Autodesk Fusion 360 part; units mm, degrees
(part 3 of 9)
  line L388 (-87.1879, -68.7148) -> (-81.5345, -68.7148) construction
  line L389 (-81.5345, -68.7148) -> (-81.5345, -58.1314) construction
  line L390 (-81.5345, -58.1314) -> (-87.1879, -58.1314) construction
  line L391 (-87.1879, -58.1314) -> (-87.1879, -68.7148) construction
  line L392 (-70.5192, -68.7148) -> (-65.7856, -68.7148) construction
  line L393 (-65.7856, -68.7148) -> (-65.7856, -58.1314) construction
  line L394 (-65.7856, -58.1314) -> (-70.5192, -58.1314) construction
  line L395 (-70.5192, -58.1314) -> (-70.5192, -68.7148) construction
  line L396 (-53.8504, -68.7148) -> (-48.7396, -68.7148) construction
  line L397 (-48.7396, -68.7148) -> (-48.7396, -58.1314) construction
  line L398 (-48.7396, -58.1314) -> (-53.8504, -58.1314) construction
  line L399 (-53.8504, -58.1314) -> (-53.8504, -68.7148) construction
  line L400 (-37.1817, -68.7148) -> (-30.2519, -68.7148) construction
  line L401 (-30.2519, -68.7148) -> (-30.2519, -58.1314) construction
  line L402 (-30.2519, -58.1314) -> (-37.1817, -58.1314) construction
  line L403 (-37.1817, -58.1314) -> (-37.1817, -68.7148) construction
  line L404 (-17.0129, -68.7148) -> (-16.0104, -68.7148) construction
  line L405 (-16.0104, -68.7148) -> (-16.0104, -58.1314) construction
  line L406 (-16.0104, -58.1314) -> (-17.0129, -58.1314) construction
  line L407 (-17.0129, -58.1314) -> (-17.0129, -68.7148) construction
  line L408 (-3.8442, -68.7148) -> (1.8092, -68.7148) construction
  line L409 (1.8092, -68.7148) -> (1.8092, -58.1314) construction
  line L410 (1.8092, -58.1314) -> (-3.8442, -58.1314) construction
  line L411 (-3.8442, -58.1314) -> (-3.8442, -68.7148) construction
  line L412 (12.8246, -68.7148) -> (19.5012, -68.7148) construction
  line L413 (19.5012, -68.7148) -> (19.5012, -58.1314) construction
  line L414 (19.5012, -58.1314) -> (12.8246, -58.1314) construction
  line L415 (12.8246, -58.1314) -> (12.8246, -68.7148) construction
  line L416 (29.4933, -68.7148) -> (36.5833, -68.7148) construction
  line L417 (36.5833, -68.7148) -> (36.5833, -58.1314) construction
  line L418 (36.5833, -58.1314) -> (29.4933, -58.1314) construction
  line L419 (29.4933, -58.1314) -> (29.4933, -68.7148) construction
  line L420 (46.1621, -68.7148) -> (52.8593, -68.7148) construction
  line L421 (52.8593, -68.7148) -> (52.8593, -58.1314) construction
  line L422 (52.8593, -58.1314) -> (46.1621, -58.1314) construction
  line L423 (46.1621, -58.1314) -> (46.1621, -68.7148) construction
  line L424 (62.8308, -68.7148) -> (68.7736, -68.7148) construction
  line L425 (68.7736, -68.7148) -> (68.7736, -58.1314) construction
  line L426 (68.7736, -58.1314) -> (62.8308, -58.1314) construction
  line L427 (62.8308, -58.1314) -> (62.8308, -68.7148) construction
  line L428 (79.4996, -68.7148) -> (85.5044, -68.7148) construction
  line L429 (85.5044, -68.7148) -> (85.5044, -58.1314) construction
  line L430 (85.5044, -58.1314) -> (79.4996, -58.1314) construction
  line L431 (79.4996, -58.1314) -> (79.4996, -68.7148) construction
  line L432 (96.1683, -68.7148) -> (102.5183, -68.7148) construction
  line L433 (102.5183, -68.7148) -> (102.5183, -58.1314) construction
  line L434 (102.5183, -58.1314) -> (96.1683, -58.1314) construction
  line L435 (96.1683, -58.1314) -> (96.1683, -68.7148) construction
  line L436 (-87.1879, -87.2148) -> (-81.1573, -87.2148) construction
  line L437 (-81.1573, -87.2148) -> (-81.1573, -76.6314) construction
  line L438 (-81.1573, -76.6314) -> (-87.1879, -76.6314) construction
  line L439 (-87.1879, -76.6314) -> (-87.1879, -87.2148) construction
  line L440 (-70.5192, -87.2148) -> (-64.8658, -87.2148) construction
  line L441 (-64.8658, -87.2148) -> (-64.8658, -76.6314) construction
  line L442 (-64.8658, -76.6314) -> (-70.5192, -76.6314) construction
  line L443 (-70.5192, -76.6314) -> (-70.5192, -87.2148) construction
  line L444 (-53.8504, -87.2148) -> (-47.1532, -87.2148) construction
  line L445 (-47.1532, -87.2148) -> (-47.1532, -76.6314) construction
  line L446 (-47.1532, -76.6314) -> (-53.8504, -76.6314) construction
  line L447 (-53.8504, -76.6314) -> (-53.8504, -87.2148) construction
  line L448 (-37.1817, -87.2148) -> (-31.2389, -87.2148) construction
  line L449 (-31.2389, -87.2148) -> (-31.2389, -76.6314) construction
  line L450 (-31.2389, -76.6314) -> (-37.1817, -76.6314) construction
  line L451 (-37.1817, -76.6314) -> (-37.1817, -87.2148) construction
  line L452 (-20.5129, -87.2148) -> (-14.4823, -87.2148) construction
  line L453 (-14.4823, -87.2148) -> (-14.4823, -76.6314) construction
  line L454 (-14.4823, -76.6314) -> (-20.5129, -76.6314) construction
  line L455 (-20.5129, -76.6314) -> (-20.5129, -87.2148) construction
  line L456 (-0.3442, -87.2148) -> (0.6584, -87.2148) construction
  line L457 (0.6584, -87.2148) -> (0.6584, -76.6314) construction
  line L458 (0.6584, -76.6314) -> (-0.3442, -76.6314) construction
  line L459 (-0.3442, -76.6314) -> (-0.3442, -87.2148) construction
  line L460 (12.8246, -87.2148) -> (18.7829, -87.2148) construction
  line L461 (18.7829, -87.2148) -> (18.7829, -76.6314) construction
  line L462 (18.7829, -76.6314) -> (12.8246, -76.6314) construction
  line L463 (12.8246, -76.6314) -> (12.8246, -87.2148) construction
  line L464 (29.4933, -87.2148) -> (35.4361, -87.2148) construction
  line L465 (35.4361, -87.2148) -> (35.4361, -76.6314) construction
  line L466 (35.4361, -76.6314) -> (29.4933, -76.6314) construction
  line L467 (29.4933, -76.6314) -> (29.4933, -87.2148) construction
  line L468 (46.1621, -87.2148) -> (52.8387, -87.2148) construction
  line L469 (52.8387, -87.2148) -> (52.8387, -76.6314) construction
  line L470 (52.8387, -76.6314) -> (46.1621, -76.6314) construction
  line L471 (46.1621, -76.6314) -> (46.1621, -87.2148) construction
  line L472 (62.8308, -87.2148) -> (69.7761, -87.2148) construction
  line L473 (69.7761, -87.2148) -> (69.7761, -76.6314) construction
  line L474 (69.7761, -76.6314) -> (62.8308, -76.6314) construction
  line L475 (62.8308, -76.6314) -> (62.8308, -87.2148) construction
  line L476 (79.4996, -87.2148) -> (85.153, -87.2148) construction
  line L477 (85.153, -87.2148) -> (85.153, -76.6314) construction
  line L478 (85.153, -76.6314) -> (79.4996, -76.6314) construction
  line L479 (79.4996, -76.6314) -> (79.4996, -87.2148) construction
  line L480 (96.1683, -87.2148) -> (102.5183, -87.2148) construction
  line L481 (102.5183, -87.2148) -> (102.5183, -76.6314) construction
  line L482 (102.5183, -76.6314) -> (96.1683, -76.6314) construction
  line L483 (96.1683, -76.6314) -> (96.1683, -87.2148) construction
extrude "Extrude3" add 1 faces at (-13.7, 108.5, 5) along direction (0, 0, 1) blind 2
sketch "Sketch11" plane through (0, 0, 0) normal (0, 0, 1) x (1, 0, 0)
  line L0 (-86.6667, 80) -> (-81.3249, 80) construction
  line L1 (-81.3249, 80) -> (-81.3249, 90) construction
  line L2 (-81.3249, 90) -> (-86.6667, 90) construction
  line L3 (-86.6667, 90) -> (-86.6667, 80) construction
  line L4 (-70, 80) -> (-64.3018, 80) construction
  line L5 (-64.3018, 80) -> (-64.3018, 90) construction
  line L6 (-64.3018, 90) -> (-70, 90) construction
  line L7 (-70, 90) -> (-70, 80) construction
  line L8 (-53.3333, 80) -> (-47.4153, 80) construction
  line L9 (-47.4153, 80) -> (-47.4153, 90) construction
  line L10 (-47.4153, 90) -> (-53.3333, 90) construction
  line L11 (-53.3333, 90) -> (-53.3333, 80) construction
  line L12 (-36.6667, 80) -> (-35.7194, 80) construction
  line L13 (-35.7194, 80) -> (-35.7194, 90) construction
  line L14 (-35.7194, 90) -> (-36.6667, 90) construction
  line L15 (-36.6667, 90) -> (-36.6667, 80) construction
  line L16 (-20, 80) -> (-14.3018, 80) construction
  line L17 (-14.3018, 80) -> (-14.3018, 90) construction
  line L18 (-14.3018, 90) -> (-20, 90) construction
  line L19 (-20, 90) -> (-20, 80) construction
  line L20 (-3.3333, 80) -> (2.3405, 80) construction
  line L21 (2.3405, 80) -> (2.3405, 90) construction
  line L22 (2.3405, 90) -> (-3.3333, 90) construction
  line L23 (-3.3333, 90) -> (-3.3333, 80) construction
  line L24 (13.3333, 80) -> (19.6419, 80) construction
  line L25 (19.6419, 80) -> (19.6419, 90) construction
  line L26 (19.6419, 90) -> (13.3333, 90) construction
  line L27 (13.3333, 90) -> (13.3333, 80) construction
  line L28 (30, 80) -> (34.8291, 80) construction
  line L29 (34.8291, 80) -> (34.8291, 90) construction
  line L30 (34.8291, 90) -> (30, 90) construction
  line L31 (30, 90) -> (30, 80) construction
  line L32 (46.6667, 80) -> (52.2966, 80) construction
  line L33 (52.2966, 80) -> (52.2966, 90) construction
  line L34 (52.2966, 90) -> (46.6667, 90) construction
  line L35 (46.6667, 90) -> (46.6667, 80) construction
  line L36 (63.3333, 80) -> (68.9729, 80) construction
  line L37 (68.9729, 80) -> (68.9729, 90) construction
  line L38 (68.9729, 90) -> (63.3333, 90) construction
  line L39 (63.3333, 90) -> (63.3333, 80) construction
  line L40 (80, 80) -> (84.8291, 80) construction
  line L41 (84.8291, 80) -> (84.8291, 90) construction
  line L42 (84.8291, 90) -> (80, 90) construction
  line L43 (80, 90) -> (80, 80) construction
  line L44 (-86.6667, 60) -> (-81.0075, 60) construction
  line L45 (-81.0075, 60) -> (-81.0075, 70) construction
  line L46 (-81.0075, 70) -> (-86.6667, 70) construction
  line L47 (-86.6667, 70) -> (-86.6667, 60) construction
  line L48 (-70, 60) -> (-64.6582, 60) construction
  line L49 (-64.6582, 60) -> (-64.6582, 70) construction
  line L50 (-64.6582, 70) -> (-70, 70) construction
  line L51 (-70, 70) -> (-70, 60) construction
  line L52 (-53.3333, 60) -> (-47.7181, 60) construction
  line L53 (-47.7181, 60) -> (-47.7181, 70) construction
  line L54 (-47.7181, 70) -> (-53.3333, 70) construction
  line L55 (-53.3333, 70) -> (-53.3333, 60) construction
  line L56 (-36.6667, 60) -> (-31.0271, 60) construction
  line L57 (-31.0271, 60) -> (-31.0271, 70) construction
  line L58 (-31.0271, 70) -> (-36.6667, 70) construction
  line L59 (-36.6667, 70) -> (-36.6667, 60) construction
  line L60 (-20, 60) -> (-14.3408, 60) construction
  line L61 (-14.3408, 60) -> (-14.3408, 70) construction
  line L62 (-14.3408, 70) -> (-20, 70) construction
  line L63 (-20, 70) -> (-20, 60) construction
  line L64 (-3.3333, 60) -> (5.8708, 60) construction
  line L65 (5.8708, 60) -> (5.8708, 70) construction
  line L66 (5.8708, 70) -> (-3.3333, 70) construction
  line L67 (-3.3333, 70) -> (-3.3333, 60) construction
  line L68 (13.3333, 60) -> (20.0325, 60) construction
  line L69 (20.0325, 60) -> (20.0325, 70) construction
  line L70 (20.0325, 70) -> (13.3333, 70) construction
  line L71 (13.3333, 70) -> (13.3333, 60) construction
  line L72 (30, 60) -> (35.6396, 60) construction
  line L73 (35.6396, 60) -> (35.6396, 70) construction
  line L74 (35.6396, 70) -> (30, 70) construction
  line L75 (30, 70) -> (30, 60) construction
  line L76 (46.6667, 60) -> (52.3259, 60) construction
  line L77 (52.3259, 60) -> (52.3259, 70) construction
  line L78 (52.3259, 70) -> (46.6667, 70) construction
  line L79 (46.6667, 70) -> (46.6667, 60) construction
  line L80 (63.3333, 60) -> (64.2806, 60) construction
  line L81 (64.2806, 60) -> (64.2806, 70) construction
  line L82 (64.2806, 70) -> (63.3333, 70) construction
  line L83 (63.3333, 70) -> (63.3333, 60) construction
  line L84 (80, 60) -> (86.6211, 60) construction
  line L85 (86.6211, 60) -> (86.6211, 70) construction
  line L86 (86.6211, 70) -> (80, 70) construction
  line L87 (80, 70) -> (80, 60) construction
  line L88 (-86.6667, 40) -> (-80.7487, 40) construction
  line L89 (-80.7487, 40) -> (-80.7487, 50) construction
  line L90 (-80.7487, 50) -> (-86.6667, 50) construction
  line L91 (-86.6667, 50) -> (-86.6667, 40) construction
  line L92 (-70, 40) -> (-63.6914, 40) construction
  line L93 (-63.6914, 40) -> (-63.6914, 50) construction
  line L94 (-63.6914, 50) -> (-70, 50) construction
  line L95 (-70, 50) -> (-70, 40) construction
  line L96 (-53.3333, 40) -> (-47.9915, 40) construction
  line L97 (-47.9915, 40) -> (-47.9915, 50) construction
  line L98 (-47.9915, 50) -> (-53.3333, 50) construction
  line L99 (-53.3333, 50) -> (-53.3333, 40) construction
  line L100 (-36.6667, 40) -> (-35.7194, 40) construction
  line L101 (-35.7194, 40) -> (-35.7194, 50) construction
  line L102 (-35.7194, 50) -> (-36.6667, 50) construction
  line L103 (-36.6667, 50) -> (-36.6667, 40) construction
  line L104 (-20, 40) -> (-13.4521, 40) construction
  line L105 (-13.4521, 40) -> (-13.4521, 50) construction
  line L106 (-13.4521, 50) -> (-20, 50) construction
  line L107 (-20, 50) -> (-20, 40) construction
  line L108 (-3.3333, 40) -> (-2.386, 40) construction
  line L109 (-2.386, 40) -> (-2.386, 50) construction
  line L110 (-2.386, 50) -> (-3.3333, 50) construction
  line L111 (-3.3333, 50) -> (-3.3333, 40) construction
  line L112 (13.3333, 40) -> (18.6751, 40) construction
  line L113 (18.6751, 40) -> (18.6751, 50) construction
  line L114 (18.6751, 50) -> (13.3333, 50) construction
  line L115 (13.3333, 50) -> (13.3333, 40) construction
  line L116 (30, 40) -> (36.3086, 40) construction
  line L117 (36.3086, 40) -> (36.3086, 50) construction
  line L118 (36.3086, 50) -> (30, 50) construction
  line L119 (30, 50) -> (30, 40) construction
  line L120 (46.6667, 40) -> (52.3405, 40) construction
  line L121 (52.3405, 40) -> (52.3405, 50) construction
  line L122 (52.3405, 50) -> (46.6667, 50) construction
  line L123 (46.6667, 50) -> (46.6667, 40) construction
  line L124 (63.3333, 40) -> (68.6751, 40) construction
  line L125 (68.6751, 40) -> (68.6751, 50) construction
  line L126 (68.6751, 50) -> (63.3333, 50) construction
  line L127 (63.3333, 50) -> (63.3333, 40) construction
  line L128 (80, 40) -> (84.4727, 40) construction
  line L129 (84.4727, 40) -> (84.4727, 50) construction
  line L130 (84.4727, 50) -> (80, 50) construction
  line L131 (80, 50) -> (80, 40) construction
  line L132 (-86.6667, 20) -> (-80.9929, 20) construction
  line L133 (-80.9929, 20) -> (-80.9929, 30) construction
  line L134 (-80.9929, 30) -> (-86.6667, 30) construction
  line L135 (-86.6667, 30) -> (-86.6667, 20) construction
  line L136 (-70, 20) -> (-63.3789, 20) construction
  line L137 (-63.3789, 20) -> (-63.3789, 30) construction
  line L138 (-63.3789, 30) -> (-70, 30) construction
  line L139 (-70, 30) -> (-70, 20) construction
  line L140 (-53.3333, 20) -> (-47.6937, 20) construction
  line L141 (-47.6937, 20) -> (-47.6937, 30) construction
  line L142 (-47.6937, 30) -> (-53.3333, 30) construction
  line L143 (-53.3333, 30) -> (-53.3333, 20) construction
  line L144 (-36.6667, 20) -> (-29.9675, 20) construction
  line L145 (-29.9675, 20) -> (-29.9675, 30) construction
  line L146 (-29.9675, 30) -> (-36.6667, 30) construction
  line L147 (-36.6667, 30) -> (-36.6667, 20) construction
  line L148 (-20, 20) -> (-13.6719, 20) construction
  line L149 (-13.6719, 20) -> (-13.6719, 30) construction
  line L150 (-13.6719, 30) -> (-20, 30) construction
  line L151 (-20, 30) -> (-20, 20) construction
  line L152 (-3.3333, 20) -> (2.2819, 20) construction
  line L153 (2.2819, 20) -> (2.2819, 30) construction
  line L154 (2.2819, 30) -> (-3.3333, 30) construction
  line L155 (-3.3333, 30) -> (-3.3333, 20) construction
  line L156 (13.3333, 20) -> (19.8812, 20) construction
  line L157 (19.8812, 20) -> (19.8812, 30) construction
  line L158 (19.8812, 30) -> (13.3333, 30) construction
  line L159 (13.3333, 30) -> (13.3333, 20) construction
  line L160 (30, 20) -> (36.8457, 20) construction
  line L161 (36.8457, 20) -> (36.8457, 30) construction
  line L162 (36.8457, 30) -> (30, 30) construction
  line L163 (30, 30) -> (30, 20) construction
  line L164 (46.6667, 20) -> (52.9753, 20) construction
  line L165 (52.9753, 20) -> (52.9753, 30) construction
  line L166 (52.9753, 30) -> (46.6667, 30) construction
  line L167 (46.6667, 30) -> (46.6667, 20) construction
  line L168 (63.3333, 20) -> (68.9632, 20) construction
  line L169 (68.9632, 20) -> (68.9632, 30) construction
  line L170 (68.9632, 30) -> (63.3333, 30) construction
  line L171 (63.3333, 30) -> (63.3333, 20) construction
  line L172 (80, 20) -> (86.8311, 20) construction
  line L173 (86.8311, 20) -> (86.8311, 30) construction
  line L174 (86.8311, 30) -> (80, 30) construction
  line L175 (80, 30) -> (80, 20) construction
  line L176 (-86.6667, 0) -> (-81.0515, 0) construction
  line L177 (-81.0515, 0) -> (-81.0515, 10) construction
  line L178 (-81.0515, 10) -> (-86.6667, 10) construction
  line L179 (-86.6667, 10) -> (-86.6667, 0) construction
  line L180 (-70, 0) -> (-63.3008, 0) construction
  line L181 (-63.3008, 0) -> (-63.3008, 10) construction
  line L182 (-63.3008, 10) -> (-70, 10) construction
  line L183 (-70, 10) -> (-70, 0) construction
  line L184 (-53.3333, 0) -> (-48.8606, 0) construction
  line L185 (-48.8606, 0) -> (-48.8606, 10) construction
  line L186 (-48.8606, 10) -> (-53.3333, 10) construction
  line L187 (-53.3333, 10) -> (-53.3333, 0) construction
  line L188 (-36.6667, 0) -> (-31.2614, 0) construction
  line L189 (-31.2614, 0) -> (-31.2614, 10) construction
  line L190 (-31.2614, 10) -> (-36.6667, 10) construction
  line L191 (-36.6667, 10) -> (-36.6667, 0) construction
  line L192 (-20, 0) -> (-13.3789, 0) construction
  line L193 (-13.3789, 0) -> (-13.3789, 10) construction
  line L194 (-13.3789, 10) -> (-20, 10) construction
  line L195 (-20, 10) -> (-20, 0) construction
  line L196 (-3.3333, 0) -> (2.3259, 0) construction
  line L197 (2.3259, 0) -> (2.3259, 10) construction
  line L198 (2.3259, 10) -> (-3.3333, 10) construction
  line L199 (-3.3333, 10) -> (-3.3333, 0) construction
  line L200 (13.3333, 0) -> (22.5374, 0) construction
  line L201 (22.5374, 0) -> (22.5374, 10) construction
  line L202 (22.5374, 10) -> (13.3333, 10) construction
  line L203 (13.3333, 10) -> (13.3333, 0) construction
  line L204 (30, 0) -> (36.8457, 0) construction
  line L205 (36.8457, 0) -> (36.8457, 10) construction
  line L206 (36.8457, 10) -> (30, 10) construction
  line L207 (30, 10) -> (30, 0) construction
  line L208 (46.6667, 0) -> (51.1394, 0) construction
  line L209 (51.1394, 0) -> (51.1394, 10) construction
  line L210 (51.1394, 10) -> (46.6667, 10) construction
  line L211 (46.6667, 10) -> (46.6667, 0) construction
  line L212 (63.3333, 0) -> (68.1624, 0) construction
  line L213 (68.1624, 0) -> (68.1624, 10) construction
  line L214 (68.1624, 10) -> (63.3333, 10) construction
  line L215 (63.3333, 10) -> (63.3333, 0) construction
  line L216 (80, 0) -> (83.9551, 0) construction
  line L217 (83.9551, 0) -> (83.9551, 10) construction
  line L218 (83.9551, 10) -> (80, 10) construction
  line L219 (80, 10) -> (80, 0) construction
  line L220 (-86.6667, -20) -> (-81.0075, -20) construction
  line L221 (-81.0075, -20) -> (-81.0075, -10) construction
  line L222 (-81.0075, -10) -> (-86.6667, -10) construction
  line L223 (-86.6667, -10) -> (-86.6667, -20) construction
  line L224 (-70, -20) -> (-60.7959, -20) construction
  line L225 (-60.7959, -20) -> (-60.7959, -10) construction
  line L226 (-60.7959, -10) -> (-70, -10) construction
  line L227 (-70, -10) -> (-70, -20) construction
  line L228 (-53.3333, -20) -> (-47.9915, -20) construction
  line L229 (-47.9915, -20) -> (-47.9915, -10) construction
  line L230 (-47.9915, -10) -> (-53.3333, -10) construction
  line L231 (-53.3333, -10) -> (-53.3333, -20) construction
  line L232 (-36.6667, -20) -> (-35.7194, -20) construction
  line L233 (-35.7194, -20) -> (-35.7194, -10) construction
  line L234 (-35.7194, -10) -> (-36.6667, -10) construction
  line L235 (-36.6667, -10) -> (-36.6667, -20) construction
  line L236 (-20, -20) -> (-14.3604, -20) construction
  line L237 (-14.3604, -20) -> (-14.3604, -10) construction
  line L238 (-14.3604, -10) -> (-20, -10) construction
  line L239 (-20, -10) -> (-20, -20) construction
  line L240 (-3.3333, -20) -> (2.3649, -20) construction
  line L241 (2.3649, -20) -> (2.3649, -10) construction
  line L242 (2.3649, -10) -> (-3.3333, -10) construction
  line L243 (-3.3333, -10) -> (-3.3333, -20) construction
  line L244 (13.3333, -20) -> (14.2806, -20) construction
  line L245 (14.2806, -20) -> (14.2806, -10) construction
  line L246 (14.2806, -10) -> (13.3333, -10) construction
  line L247 (13.3333, -10) -> (13.3333, -20) construction
  line L248 (30, -20) -> (35.3418, -20) construction
  line L249 (35.3418, -20) -> (35.3418, -10) construction
  line L250 (35.3418, -10) -> (30, -10) construction
  line L251 (30, -10) -> (30, -20) construction
  line L252 (46.6667, -20) -> (52.072, -20) construction
  line L253 (52.072, -20) -> (52.072, -10) construction
  line L254 (52.072, -10) -> (46.6667, -10) construction
  line L255 (46.6667, -10) -> (46.6667, -20) construction
  line L256 (63.3333, -20) -> (68.6751, -20) construction
  line L257 (68.6751, -20) -> (68.6751, -10) construction
  line L258 (68.6751, -10) -> (63.3333, -10) construction
  line L259 (63.3333, -10) -> (63.3333, -20) construction
  line L260 (80, -20) -> (85.6396, -20) construction
  line L261 (85.6396, -20) -> (85.6396, -10) construction
  line L262 (85.6396, -10) -> (80, -10) construction
  line L263 (80, -10) -> (80, -20) construction
  line L264 (-86.6667, -40) -> (-80.7487, -40) construction
  line L265 (-80.7487, -40) -> (-80.7487, -30) construction
  line L266 (-80.7487, -30) -> (-86.6667, -30) construction
  line L267 (-86.6667, -30) -> (-86.6667, -40) construction
  line L268 (-70, -40) -> (-64.082, -40) construction
  line L269 (-64.082, -40) -> (-64.082, -30) construction
  line L270 (-64.082, -30) -> (-70, -30) construction
  line L271 (-70, -30) -> (-70, -40) construction
  line L272 (-53.3333, -40) -> (-47.0247, -40) construction
  line L273 (-47.0247, -40) -> (-47.0247, -30) construction
  line L274 (-47.0247, -30) -> (-53.3333, -30) construction
  line L275 (-53.3333, -30) -> (-53.3333, -40) construction
  line L276 (-36.6667, -40) -> (-31.3249, -40) construction
  line L277 (-31.3249, -40) -> (-31.3249, -30) construction
  line L278 (-31.3249, -30) -> (-36.6667, -30) construction
  line L279 (-36.6667, -30) -> (-36.6667, -40) construction
  line L280 (-20, -40) -> (-19.0527, -40) construction
  line L281 (-19.0527, -40) -> (-19.0527, -30) construction
  line L282 (-19.0527, -30) -> (-20, -30) construction
  line L283 (-20, -30) -> (-20, -40) construction
  line L284 (-3.3333, -40) -> (2.9753, -40) construction
  line L285 (2.9753, -40) -> (2.9753, -30) construction
  line L286 (2.9753, -30) -> (-3.3333, -30) construction
  line L287 (-3.3333, -30) -> (-3.3333, -40) construction
  line L288 (13.3333, -40) -> (18.9485, -40) construction
  line L289 (18.9485, -40) -> (18.9485, -30) construction
  line L290 (18.9485, -30) -> (13.3333, -30) construction
  line L291 (13.3333, -30) -> (13.3333, -40) construction
  line L292 (30, -40) -> (34.8291, -40) construction
  line L293 (34.8291, -40) -> (34.8291, -30) construction
  line L294 (34.8291, -30) -> (30, -30) construction
  line L295 (30, -30) -> (30, -40) construction
  line L296 (46.6667, -40) -> (52.2966, -40) construction
  line L297 (52.2966, -40) -> (52.2966, -30) construction
  line L298 (52.2966, -30) -> (46.6667, -30) construction
  line L299 (46.6667, -30) -> (46.6667, -40) construction
  line L300 (63.3333, -40) -> (68.9729, -40) construction
  line L301 (68.9729, -40) -> (68.9729, -30) construction
  line L302 (68.9729, -30) -> (63.3333, -30) construction
  line L303 (63.3333, -30) -> (63.3333, -40) construction
  line L304 (80, -40) -> (84.8291, -40) construction
  line L305 (84.8291, -40) -> (84.8291, -30) construction
  line L306 (84.8291, -30) -> (80, -30) construction
  line L307 (80, -30) -> (80, -40) construction
  line L308 (-86.6667, -60) -> (-81.3249, -60) construction
  line L309 (-81.3249, -60) -> (-81.3249, -50) construction
  line L310 (-81.3249, -50) -> (-86.6667, -50) construction
  line L311 (-86.6667, -50) -> (-86.6667, -60) construction
  line L312 (-70, -60) -> (-65.5273, -60) construction
  line L313 (-65.5273, -60) -> (-65.5273, -50) construction
  line L314 (-65.5273, -50) -> (-70, -50) construction
  line L315 (-70, -50) -> (-70, -60) construction
  line L316 (-53.3333, -60) -> (-48.5042, -60) construction
  line L317 (-48.5042, -60) -> (-48.5042, -50) construction
  line L318 (-48.5042, -50) -> (-53.3333, -50) construction
  line L319 (-53.3333, -50) -> (-53.3333, -60) construction
  line L320 (-36.6667, -60) -> (-31.0271, -60) construction
  line L321 (-31.0271, -60) -> (-31.0271, -50) construction
  line L322 (-31.0271, -50) -> (-36.6667, -50) construction
  line L323 (-36.6667, -50) -> (-36.6667, -60) construction
  line L324 (-20, -60) -> (-14.6582, -60) construction
  line L325 (-14.6582, -60) -> (-14.6582, -50) construction
  line L326 (-14.6582, -50) -> (-20, -50) construction
  line L327 (-20, -50) -> (-20, -60) construction
  line L328 (-3.3333, -60) -> (2.2966, -60) construction
  line L329 (2.2966, -60) -> (2.2966, -50) construction
  line L330 (2.2966, -50) -> (-3.3333, -50) construction
  line L331 (-3.3333, -50) -> (-3.3333, -60) construction
  line L332 (13.3333, -60) -> (18.9729, -60) construction
  line L333 (18.9729, -60) -> (18.9729, -50) construction
  line L334 (18.9729, -50) -> (13.3333, -50) construction
  line L335 (13.3333, -50) -> (13.3333, -60) construction
  line L336 (30, -60) -> (36.5479, -60) construction
  line L337 (36.5479, -60) -> (36.5479, -50) construction
  line L338 (36.5479, -50) -> (30, -50) construction
  line L339 (30, -50) -> (30, -60) construction
  line L340 (46.6667, -60) -> (47.614, -60) construction
  line L341 (47.614, -60) -> (47.614, -50) construction
  line L342 (47.614, -50) -> (46.6667, -50) construction
  line L343 (46.6667, -50) -> (46.6667, -60) construction
  line L344 (63.3333, -60) -> (68.6751, -60) construction
  line L345 (68.6751, -60) -> (68.6751, -50) construction
  line L346 (68.6751, -50) -> (63.3333, -50) construction
  line L347 (63.3333, -50) -> (63.3333, -60) construction
  line L348 (80, -60) -> (86.3086, -60) construction
  line L349 (86.3086, -60) -> (86.3086, -50) construction
  line L350 (86.3086, -50) -> (80, -50) construction
  line L351 (80, -50) -> (80, -60) construction
  line L352 (-86.6667, -80) -> (-81.0271, -80) construction
  line L353 (-81.0271, -80) -> (-81.0271, -70) construction
  line L354 (-81.0271, -70) -> (-86.6667, -70) construction
  line L355 (-86.6667, -70) -> (-86.6667, -80) construction
  line L356 (-70, -80) -> (-63.3008, -80) construction
  line L357 (-63.3008, -80) -> (-63.3008, -70) construction
  line L358 (-63.3008, -70) -> (-70, -70) construction
  line L359 (-70, -70) -> (-70, -80) construction
  line L360 (-53.3333, -80) -> (-47.0052, -80) construction
  line L361 (-47.0052, -80) -> (-47.0052, -70) construction
  line L362 (-47.0052, -70) -> (-53.3333, -70) construction
  line L363 (-53.3333, -70) -> (-53.3333, -80) construction
  line L364 (-36.6667, -80) -> (-31.0515, -80) construction
  line L365 (-31.0515, -80) -> (-31.0515, -70) construction
  line L366 (-31.0515, -70) -> (-36.6667, -70) construction
  line L367 (-36.6667, -70) -> (-36.6667, -80) construction
  line L368 (-20, -80) -> (-14.3262, -80) construction
  line L369 (-14.3262, -80) -> (-14.3262, -70) construction
  line L370 (-14.3262, -70) -> (-20, -70) construction
  line L371 (-20, -70) -> (-20, -80) construction
  line L372 (-3.3333, -80) -> (2.3259, -80) construction
  line L373 (2.3259, -80) -> (2.3259, -70) construction
  line L374 (2.3259, -70) -> (-3.3333, -70) construction
  line L375 (-3.3333, -70) -> (-3.3333, -80) construction
  line L376 (13.3333, -80) -> (18.6751, -80) construction
  line L377 (18.6751, -80) -> (18.6751, -70) construction
  line L378 (18.6751, -70) -> (13.3333, -70) construction
  line L379 (13.3333, -70) -> (13.3333, -80) construction
  line L380 (30, -80) -> (35.6152, -80) construction
  line L381 (35.6152, -80) -> (35.6152, -70) construction
  line L382 (35.6152, -70) -> (30, -70) construction
  line L383 (30, -70) -> (30, -80) construction
  line L384 (46.6667, -80) -> (52.3063, -80) construction
  line L385 (52.3063, -80) -> (52.3063, -70) construction
  line L386 (52.3063, -70) -> (46.6667, -70) construction
  line L387 (46.6667, -70) -> (46.6667, -80) construction
  line L388 (63.3333, -80) -> (68.7386, -80) construction
  line L389 (68.7386, -80) -> (68.7386, -70) construction
  line L390 (68.7386, -70) -> (63.3333, -70) construction
  line L391 (63.3333, -70) -> (63.3333, -80) construction
  line L392 (80, -80) -> (86.5625, -80) construction
  line L393 (86.5625, -80) -> (86.5625, -70) construction
  line L394 (86.5625, -70) -> (80, -70) construction
  line L395 (80, -70) -> (80, -80) construction
  line L396 (-86.6667, -100) -> (-81.0368, -100) construction
  line L397 (-81.0368, -100) -> (-81.0368, -90) construction
  line L398 (-81.0368, -90) -> (-86.6667, -90) construction
  line L399 (-86.6667, -90) -> (-86.6667, -100) construction
  line L400 (-70, -100) -> (-64.3018, -100) construction
  line L401 (-64.3018, -100) -> (-64.3018, -90) construction
  line L402 (-64.3018, -90) -> (-70, -90) construction
  line L403 (-70, -90) -> (-70, -100) construction
  line L404 (-53.3333, -100) -> (-47.9915, -100) construction
  line L405 (-47.9915, -100) -> (-47.9915, -90) construction
  line L406 (-47.9915, -90) -> (-53.3333, -90) construction
  line L407 (-53.3333, -90) -> (-53.3333, -100) construction
  line L408 (-36.6667, -100) -> (-30.3386, -100) construction
  line L409 (-30.3386, -100) -> (-30.3386, -90) construction
  line L410 (-30.3386, -90) -> (-36.6667, -90) construction
  line L411 (-36.6667, -90) -> (-36.6667, -100) construction
  line L412 (-20, -100) -> (-14.3848, -100) construction
  line L413 (-14.3848, -100) -> (-14.3848, -90) construction
  line L414 (-14.3848, -90) -> (-20, -90) construction
  line L415 (-20, -90) -> (-20, -100) construction
  line L416 (-3.3333, -100) -> (2.3649, -100) construction
  line L417 (2.3649, -100) -> (2.3649, -90) construction
  line L418 (2.3649, -90) -> (-3.3333, -90) construction
  line L419 (-3.3333, -90) -> (-3.3333, -100) construction
  line L420 (13.3333, -100) -> (18.1624, -100) construction
  line L421 (18.1624, -100) -> (18.1624, -90) construction
  line L422 (18.1624, -90) -> (13.3333, -90) construction
  line L423 (13.3333, -90) -> (13.3333, -100) construction
  line L424 (30, -100) -> (35.6299, -100) construction
  line L425 (35.6299, -100) -> (35.6299, -90) construction
  line L426 (35.6299, -90) -> (30, -90) construction
  line L427 (30, -90) -> (30, -100) construction
  line L428 (46.6667, -100) -> (52.2819, -100) construction
  line L429 (52.2819, -100) -> (52.2819, -90) construction
  line L430 (52.2819, -90) -> (46.6667, -90) construction
  line L431 (46.6667, -90) -> (46.6667, -100) construction
  line L432 (63.3333, -100) -> (69.6419, -100) construction
  line L433 (69.6419, -100) -> (69.6419, -90) construction
  line L434 (69.6419, -90) -> (63.3333, -90) construction
  line L435 (63.3333, -90) -> (63.3333, -100) construction
  line L436 (80, -100) -> (86.5625, -100) construction
  line L437 (86.5625, -100) -> (86.5625, -90) construction
  line L438 (86.5625, -90) -> (80, -90) construction
  line L439 (80, -90) -> (80, -100) construction
sketch "Sketch10" plane through (0, 0, 0) normal (0, 0, 1) x (1, 0, 0)
  line L0 (-85.9688, 87.8643) -> (-80.4342, 87.8643)
  line L1 (-80.4342, 87.8643) -> (-80.4342, 86.9341)
  line L2 (-80.4342, 86.9341) -> (-84.9662, 86.9341)
  line L3 (-84.9662, 86.9341) -> (-84.9662, 84.6293)
  line L4 (-84.9662, 84.6293) -> (-80.7753, 84.6293)
  line L5 (-80.7753, 84.6293) -> (-80.7753, 83.7508)
  line L6 (-80.7753, 83.7508) -> (-84.9662, 83.7508)
  line L7 (-84.9662, 83.7508) -> (-84.9662, 81.1773)
  line L8 (-84.9662, 81.1773) -> (-80.3567, 81.1773)
  line L9 (-80.3567, 81.1773) -> (-80.3567, 80.273)
  line L10 (-80.3567, 80.273) -> (-85.9688, 80.273)
  line L11 (-85.9688, 80.273) -> (-85.9688, 87.8643)
  spline S0 degree 3 poles (-68.7264, 82.7225) (-68.7026, 82.2915) (-68.6003, 81.9421) (-68.4215, 81.6734) knots 0 0 0 0 1 1 1 1
  spline S1 degree 3 poles (-68.4215, 81.6734) (-68.0805, 81.1701) (-67.4789, 80.9189) (-66.618, 80.9189) knots 0 0 0 0 1 1 1 1
  spline S2 degree 3 poles (-66.618, 80.9189) (-66.2325, 80.9189) (-65.8811, 80.9737) (-65.5638, 81.0843) knots 0 0 0 0 1 1 1 1
  spline S3 degree 3 poles (-65.5638, 81.0843) (-64.9509, 81.2983) (-64.644, 81.6807) (-64.644, 82.2315) knots 0 0 0 0 1 1 1 1
  spline S4 degree 3 poles (-64.644, 82.2315) (-64.644, 82.6449) (-64.7732, 82.9395) (-65.0315, 83.1152) knots 0 0 0 0 1 1 1 1
  spline S5 degree 3 poles (-65.0315, 83.1152) (-65.293, 83.2878) (-65.7033, 83.4377) (-66.2614, 83.5648) knots 0 0 0 0 1 1 1 1
  line L12 (-66.2614, 83.5648) -> (-67.2898, 83.7973)
  spline S6 degree 3 poles (-67.2898, 83.7973) (-67.9616, 83.9493) (-68.437, 84.1156) (-68.7161, 84.2986) knots 0 0 0 0 1 1 1 1
  spline S7 degree 3 poles (-68.7161, 84.2986) (-69.1987, 84.6159) (-69.4395, 85.0892) (-69.4395, 85.7197) knots 0 0 0 0 1 1 1 1
  spline S8 degree 3 poles (-69.4395, 85.7197) (-69.4395, 86.4018) (-69.2039, 86.962) (-68.7316, 87.3992) knots 0 0 0 0 1 1 1 1
  spline S9 degree 3 poles (-68.7316, 87.3992) (-68.2593, 87.8364) (-67.5916, 88.0555) (-66.7265, 88.0555) knots 0 0 0 0 1 1 1 1
  spline S10 degree 3 poles (-66.7265, 88.0555) (-65.9307, 88.0555) (-65.2548, 87.8632) (-64.6977, 87.4788) knots 0 0 0 0 1 1 1 1
  spline S11 degree 3 poles (-64.6977, 87.4788) (-64.1417, 87.0953) (-63.8637, 86.4814) (-63.8637, 85.637) knots 0 0 0 0 1 1 1 1
  line L13 (-63.8637, 85.637) -> (-64.83, 85.637)
  spline S12 degree 3 poles (-64.83, 85.637) (-64.8817, 86.0432) (-64.9923, 86.3553) (-65.1607, 86.5723) knots 0 0 0 0 1 1 1 1
  spline S13 degree 3 poles (-65.1607, 86.5723) (-65.4739, 86.9682) (-66.0062, 87.1666) (-66.7575, 87.1666) knots 0 0 0 0 1 1 1 1
  spline S14 degree 3 poles (-66.7575, 87.1666) (-67.3642, 87.1666) (-67.7993, 87.0395) (-68.0649, 86.7842) knots 0 0 0 0 1 1 1 1
  spline S15 degree 3 poles (-68.0649, 86.7842) (-68.3306, 86.5289) (-68.4629, 86.2333) (-68.4629, 85.8954) knots 0 0 0 0 1 1 1 1
  spline S16 degree 3 poles (-68.4629, 85.8954) (-68.4629, 85.5233) (-68.3078, 85.2515) (-67.9978, 85.0789) knots 0 0 0 0 1 1 1 1
  spline S17 degree 3 poles (-67.9978, 85.0789) (-67.7942, 84.9683) (-67.3342, 84.8309) (-66.618, 84.6655) knots 0 0 0 0 1 1 1 1
  line L14 (-66.618, 84.6655) -> (-65.5535, 84.4226)
  spline S18 degree 3 poles (-65.5535, 84.4226) (-65.0398, 84.3058) (-64.644, 84.1456) (-64.3649, 83.942) knots 0 0 0 0 1 1 1 1
  spline S19 degree 3 poles (-64.3649, 83.942) (-63.8823, 83.5875) (-63.6414, 83.0718) (-63.6414, 82.3969) knots 0 0 0 0 1 1 1 1
  spline S20 degree 3 poles (-63.6414, 82.3969) (-63.6414, 81.5566) (-63.9474, 80.9551) (-64.5592, 80.5934) knots 0 0 0 0 1 1 1 1
  spline S21 degree 3 poles (-64.5592, 80.5934) (-65.17, 80.2316) (-65.8811, 80.0508) (-66.6904, 80.0508) knots 0 0 0 0 1 1 1 1
  spline S22 degree 3 poles (-66.6904, 80.0508) (-67.634, 80.0508) (-68.3729, 80.2916) (-68.9073, 80.7743) knots 0 0 0 0 1 1 1 1
  spline S23 degree 3 poles (-68.9073, 80.7743) (-69.4416, 81.2528) (-69.7031, 81.9029) (-69.6928, 82.7225) knots 0 0 0 0 1 1 1 1
  line L15 (-69.6928, 82.7225) -> (-68.7264, 82.7225)
  line L16 (-52.7295, 87.8643) -> (-51.7269, 87.8643)
  line L17 (-51.7269, 87.8643) -> (-51.7269, 84.1642)
  line L18 (-51.7269, 84.1642) -> (-48.0269, 87.8643)
  line L19 (-48.0269, 87.8643) -> (-46.6058, 87.8643)
  line L20 (-46.6058, 87.8643) -> (-49.7632, 84.805)
  line L21 (-49.7632, 84.805) -> (-46.5179, 80.273)
  line L22 (-46.5179, 80.273) -> (-47.8564, 80.273)
  line L23 (-47.8564, 80.273) -> (-50.5125, 84.0815)
  line L24 (-50.5125, 84.0815) -> (-51.7269, 82.9188)
  line L25 (-51.7269, 82.9188) -> (-51.7269, 80.273)
  line L26 (-51.7269, 80.273) -> (-52.7295, 80.273)
  line L27 (-52.7295, 80.273) -> (-52.7295, 87.8643)
  line L28 (-33.7683, 87.8643) -> (-32.7296, 87.8643)
  line L29 (-32.7296, 87.8643) -> (-32.7296, 80.273)
  line L30 (-32.7296, 80.273) -> (-33.7683, 80.273)
  line L31 (-33.7683, 80.273) -> (-33.7683, 87.8643)
  spline S24 degree 3 poles (-18.7202, 82.7225) (-18.6964, 82.2915) (-18.5941, 81.9421) (-18.4153, 81.6734) knots 0 0 0 0 1 1 1 1
  spline S25 degree 3 poles (-18.4153, 81.6734) (-18.0742, 81.1701) (-17.4727, 80.9189) (-16.6118, 80.9189) knots 0 0 0 0 1 1 1 1
  spline S26 degree 3 poles (-16.6118, 80.9189) (-16.2263, 80.9189) (-15.8749, 80.9737) (-15.5576, 81.0843) knots 0 0 0 0 1 1 1 1
  spline S27 degree 3 poles (-15.5576, 81.0843) (-14.9447, 81.2983) (-14.6377, 81.6807) (-14.6377, 82.2315) knots 0 0 0 0 1 1 1 1
  spline S28 degree 3 poles (-14.6377, 82.2315) (-14.6377, 82.6449) (-14.7669, 82.9395) (-15.0253, 83.1152) knots 0 0 0 0 1 1 1 1
  spline S29 degree 3 poles (-15.0253, 83.1152) (-15.2868, 83.2878) (-15.6971, 83.4377) (-16.2552, 83.5648) knots 0 0 0 0 1 1 1 1
  line L32 (-16.2552, 83.5648) -> (-17.2836, 83.7973)
  spline S30 degree 3 poles (-17.2836, 83.7973) (-17.9553, 83.9493) (-18.4308, 84.1156) (-18.7098, 84.2986) knots 0 0 0 0 1 1 1 1
  spline S31 degree 3 poles (-18.7098, 84.2986) (-19.1925, 84.6159) (-19.4333, 85.0892) (-19.4333, 85.7197) knots 0 0 0 0 1 1 1 1
  spline S32 degree 3 poles (-19.4333, 85.7197) (-19.4333, 86.4018) (-19.1976, 86.962) (-18.7253, 87.3992) knots 0 0 0 0 1 1 1 1
  spline S33 degree 3 poles (-18.7253, 87.3992) (-18.253, 87.8364) (-17.5853, 88.0555) (-16.7203, 88.0555) knots 0 0 0 0 1 1 1 1
  spline S34 degree 3 poles (-16.7203, 88.0555) (-15.9245, 88.0555) (-15.2485, 87.8632) (-14.6915, 87.4788) knots 0 0 0 0 1 1 1 1
  spline S35 degree 3 poles (-14.6915, 87.4788) (-14.1354, 87.0953) (-13.8574, 86.4814) (-13.8574, 85.637) knots 0 0 0 0 1 1 1 1
  line L33 (-13.8574, 85.637) -> (-14.8238, 85.637)
  spline S36 degree 3 poles (-14.8238, 85.637) (-14.8754, 86.0432) (-14.986, 86.3553) (-15.1545, 86.5723) knots 0 0 0 0 1 1 1 1
  spline S37 degree 3 poles (-15.1545, 86.5723) (-15.4676, 86.9682) (-15.9999, 87.1666) (-16.7513, 87.1666) knots 0 0 0 0 1 1 1 1
  spline S38 degree 3 poles (-16.7513, 87.1666) (-17.358, 87.1666) (-17.7931, 87.0395) (-18.0587, 86.7842) knots 0 0 0 0 1 1 1 1
  spline S39 degree 3 poles (-18.0587, 86.7842) (-18.3243, 86.5289) (-18.4566, 86.2333) (-18.4566, 85.8954) knots 0 0 0 0 1 1 1 1
  spline S40 degree 3 poles (-18.4566, 85.8954) (-18.4566, 85.5233) (-18.3016, 85.2515) (-17.9915, 85.0789) knots 0 0 0 0 1 1 1 1
  spline S41 degree 3 poles (-17.9915, 85.0789) (-17.7879, 84.9683) (-17.328, 84.8309) (-16.6118, 84.6655) knots 0 0 0 0 1 1 1 1
  line L34 (-16.6118, 84.6655) -> (-15.5472, 84.4226)
  spline S42 degree 3 poles (-15.5472, 84.4226) (-15.0336, 84.3058) (-14.6377, 84.1456) (-14.3587, 83.942) knots 0 0 0 0 1 1 1 1
  spline S43 degree 3 poles (-14.3587, 83.942) (-13.876, 83.5875) (-13.6352, 83.0718) (-13.6352, 82.3969) knots 0 0 0 0 1 1 1 1
  spline S44 degree 3 poles (-13.6352, 82.3969) (-13.6352, 81.5566) (-13.9411, 80.9551) (-14.553, 80.5934) knots 0 0 0 0 1 1 1 1
  spline S45 degree 3 poles (-14.553, 80.5934) (-15.1638, 80.2316) (-15.8749, 80.0508) (-16.6841, 80.0508) knots 0 0 0 0 1 1 1 1
  spline S46 degree 3 poles (-16.6841, 80.0508) (-17.6277, 80.0508) (-18.3667, 80.2916) (-18.901, 80.7743) knots 0 0 0 0 1 1 1 1
  spline S47 degree 3 poles (-18.901, 80.7743) (-19.4354, 81.2528) (-19.6968, 81.9029) (-19.6865, 82.7225) knots 0 0 0 0 1 1 1 1
  line L35 (-19.6865, 82.7225) -> (-18.7202, 82.7225)
  spline S48 degree 3 poles (0.1831, 88.071) (1.1443, 88.071) (1.8905, 87.8177) (2.4207, 87.3113) knots 0 0 0 0 1 1 1 1
  spline S49 degree 3 poles (2.4207, 87.3113) (2.9509, 86.8049) (3.2454, 86.2292) (3.3043, 85.5853) knots 0 0 0 0 1 1 1 1
  line L36 (3.3043, 85.5853) -> (2.3018, 85.5853)
  spline S50 degree 3 poles (2.3018, 85.5853) (2.1881, 86.0742) (1.9618, 86.4618) (1.6228, 86.748) knots 0 0 0 0 1 1 1 1
  spline S51 degree 3 poles (1.6228, 86.748) (1.2828, 87.0343) (0.8063, 87.177) (0.1934, 87.177) knots 0 0 0 0 1 1 1 1
  spline S52 degree 3 poles (0.1934, 87.177) (-0.5538, 87.177) (-1.1574, 86.9144) (-1.6184, 86.3894) knots 0 0 0 0 1 1 1 1
  spline S53 degree 3 poles (-1.6184, 86.3894) (-2.0783, 85.8633) (-2.3077, 85.0582) (-2.3077, 83.973) knots 0 0 0 0 1 1 1 1
  spline S54 degree 3 poles (-2.3077, 83.973) (-2.3077, 83.0842) (-2.1, 82.3628) (-1.6845, 81.8109) knots 0 0 0 0 1 1 1 1
  spline S55 degree 3 poles (-1.6845, 81.8109) (-1.2701, 81.2579) (-0.651, 80.981) (0.1727, 80.981) knots 0 0 0 0 1 1 1 1
  spline S56 degree 3 poles (0.1727, 80.981) (0.9303, 80.981) (1.5081, 81.2724) (1.9039, 81.8543) knots 0 0 0 0 1 1 1 1
  spline S57 degree 3 poles (1.9039, 81.8543) (2.1137, 82.1612) (2.2708, 82.5643) (2.3742, 83.0635) knots 0 0 0 0 1 1 1 1
  line L37 (2.3742, 83.0635) -> (3.3767, 83.0635)
  spline S58 degree 3 poles (3.3767, 83.0635) (3.2868, 82.2646) (2.9912, 81.5938) (2.4878, 81.0533) knots 0 0 0 0 1 1 1 1
  spline S59 degree 3 poles (2.4878, 81.0533) (1.8853, 80.4022) (1.0719, 80.0766) (0.0487, 80.0766) knots 0 0 0 0 1 1 1 1
  spline S60 degree 3 poles (0.0487, 80.0766) (-0.8329, 80.0766) (-1.5739, 80.3433) (-2.1734, 80.8776) knots 0 0 0 0 1 1 1 1
  spline S61 degree 3 poles (-2.1734, 80.8776) (-2.9619, 81.5835) (-3.3568, 82.6739) (-3.3568, 84.1487) knots 0 0 0 0 1 1 1 1
  spline S62 degree 3 poles (-3.3568, 84.1487) (-3.3568, 85.268) (-3.0601, 86.1868) (-2.4679, 86.9031) knots 0 0 0 0 1 1 1 1
  spline S63 degree 3 poles (-2.4679, 86.9031) (-1.8271, 87.6813) (-0.9435, 88.071) (0.1831, 88.071) knots 0 0 0 0 1 1 1 1
  line L38 (13.6789, 87.8643) -> (14.7176, 87.8643)
  line L39 (14.7176, 87.8643) -> (14.7176, 84.7275)
  line L40 (14.7176, 84.7275) -> (18.6657, 84.7275)
  line L41 (18.6657, 84.7275) -> (18.6657, 87.8643)
  line L42 (18.6657, 87.8643) -> (19.7044, 87.8643)
  line L43 (19.7044, 87.8643) -> (19.7044, 80.273)
  line L44 (19.7044, 80.273) -> (18.6657, 80.273)
  line L45 (18.6657, 80.273) -> (18.6657, 83.8232)
  line L46 (18.6657, 83.8232) -> (14.7176, 83.8232)
  line L47 (14.7176, 83.8232) -> (14.7176, 80.273)
  line L48 (14.7176, 80.273) -> (13.6789, 80.273)
  line L49 (13.6789, 80.273) -> (13.6789, 87.8643)
  line L50 (31.438, 87.8643) -> (31.438, 83.172)
  spline S64 degree 3 poles (31.438, 83.172) (31.438, 82.6212) (31.5414, 82.1623) (31.7481, 81.7974) knots 0 0 0 0 1 1 1 1
  spline S65 degree 3 poles (31.7481, 81.7974) (32.055, 81.2466) (32.5718, 80.9706) (33.2984, 80.9706) knots 0 0 0 0 1 1 1 1
  spline S66 degree 3 poles (33.2984, 80.9706) (34.1696, 80.9706) (34.7629, 81.2683) (35.076, 81.8646) knots 0 0 0 0 1 1 1 1
  spline S67 degree 3 poles (35.076, 81.8646) (35.2445, 82.1881) (35.3293, 82.6243) (35.3293, 83.172) knots 0 0 0 0 1 1 1 1
  line L51 (35.3293, 83.172) -> (35.3293, 87.8643)
  line L52 (35.3293, 87.8643) -> (36.3731, 87.8643)
  line L53 (36.3731, 87.8643) -> (36.3731, 83.601)
  spline S68 degree 3 poles (36.3731, 83.601) (36.3731, 82.6677) (36.247, 81.9494) (35.9959, 81.446) knots 0 0 0 0 1 1 1 1
  spline S69 degree 3 poles (35.9959, 81.446) (35.5339, 80.5293) (34.6626, 80.0715) (33.3811, 80.0715) knots 0 0 0 0 1 1 1 1
  spline S70 degree 3 poles (33.3811, 80.0715) (32.0995, 80.0715) (31.2292, 80.5293) (30.7714, 81.446) knots 0 0 0 0 1 1 1 1
  spline S71 degree 3 poles (30.7714, 81.446) (30.5202, 81.9494) (30.3942, 82.6677) (30.3942, 83.601) knots 0 0 0 0 1 1 1 1
  line L54 (30.3942, 83.601) -> (30.3942, 87.8643)
  line L55 (30.3942, 87.8643) -> (31.438, 87.8643)
  line L56 (47.6779, 87.8643) -> (52.9437, 87.8643)
  line L57 (52.9437, 87.8643) -> (52.9437, 86.9341)
  line L58 (52.9437, 86.9341) -> (48.7062, 86.9341)
  line L59 (48.7062, 86.9341) -> (48.7062, 84.6293)
  line L60 (48.7062, 84.6293) -> (52.4321, 84.6293)
  line L61 (52.4321, 84.6293) -> (52.4321, 83.725)
  line L62 (52.4321, 83.725) -> (48.7062, 83.725)
  line L63 (48.7062, 83.725) -> (48.7062, 80.273)
  line L64 (48.7062, 80.273) -> (47.6779, 80.273)
  line L65 (47.6779, 80.273) -> (47.6779, 87.8643)
  line L66 (64.7755, 87.8643) -> (64.7755, 83.172)
  spline S72 degree 3 poles (64.7755, 83.172) (64.7755, 82.6212) (64.8789, 82.1623) (65.0856, 81.7974) knots 0 0 0 0 1 1 1 1
  spline S73 degree 3 poles (65.0856, 81.7974) (65.3925, 81.2466) (65.9093, 80.9706) (66.6359, 80.9706) knots 0 0 0 0 1 1 1 1
  spline S74 degree 3 poles (66.6359, 80.9706) (67.5071, 80.9706) (68.1004, 81.2683) (68.4135, 81.8646) knots 0 0 0 0 1 1 1 1
  spline S75 degree 3 poles (68.4135, 81.8646) (68.582, 82.1881) (68.6668, 82.6243) (68.6668, 83.172) knots 0 0 0 0 1 1 1 1
  line L67 (68.6668, 83.172) -> (68.6668, 87.8643)
  line L68 (68.6668, 87.8643) -> (69.7106, 87.8643)
  line L69 (69.7106, 87.8643) -> (69.7106, 83.601)
  spline S76 degree 3 poles (69.7106, 83.601) (69.7106, 82.6677) (69.5845, 81.9494) (69.3334, 81.446) knots 0 0 0 0 1 1 1 1
  spline S77 degree 3 poles (69.3334, 81.446) (68.8714, 80.5293) (68.0001, 80.0715) (66.7186, 80.0715) knots 0 0 0 0 1 1 1 1
  spline S78 degree 3 poles (66.7186, 80.0715) (65.437, 80.0715) (64.5667, 80.5293) (64.1089, 81.446) knots 0 0 0 0 1 1 1 1
  spline S79 degree 3 poles (64.1089, 81.446) (63.8577, 81.9494) (63.7317, 82.6677) (63.7317, 83.601) knots 0 0 0 0 1 1 1 1
  line L70 (63.7317, 83.601) -> (63.7317, 87.8643)
  line L71 (63.7317, 87.8643) -> (64.7755, 87.8643)
  line L72 (67.2095, 89.6626) -> (68.1758, 89.6626)
  line L73 (68.1758, 89.6626) -> (68.1758, 88.5877)
  line L74 (68.1758, 88.5877) -> (67.2095, 88.5877)
  line L75 (67.2095, 88.5877) -> (67.2095, 89.6626)
  line L76 (65.5042, 89.6626) -> (66.4705, 89.6626)
  line L77 (66.4705, 89.6626) -> (66.4705, 88.5877)
  line L78 (66.4705, 88.5877) -> (65.5042, 88.5877)
  line L79 (65.5042, 88.5877) -> (65.5042, 89.6626)
  line L80 (81.0154, 87.8643) -> (86.2812, 87.8643)
  line L81 (86.2812, 87.8643) -> (86.2812, 86.9341)
  line L82 (86.2812, 86.9341) -> (82.0437, 86.9341)
  line L83 (82.0437, 86.9341) -> (82.0437, 84.6293)
  line L84 (82.0437, 84.6293) -> (85.7696, 84.6293)
  line L85 (85.7696, 84.6293) -> (85.7696, 83.725)
  line L86 (85.7696, 83.725) -> (82.0437, 83.725)
  line L87 (82.0437, 83.725) -> (82.0437, 80.273)
  line L88 (82.0437, 80.273) -> (81.0154, 80.273)
  line L89 (81.0154, 80.273) -> (81.0154, 87.8643)
  line L90 (-85.4675, 69.3641) -> (-83.2868, 62.8994)
  line L91 (-83.2868, 62.8994) -> (-81.1319, 69.3641)
  line L92 (-81.1319, 69.3641) -> (-79.9795, 69.3641)
  line L93 (-79.9795, 69.3641) -> (-82.7493, 61.7728)
  line L94 (-82.7493, 61.7728) -> (-83.8397, 61.7728)
  line L95 (-83.8397, 61.7728) -> (-86.6044, 69.3641)
  line L96 (-86.6044, 69.3641) -> (-85.4675, 69.3641)
  line L97 (-67.1058, 69.3641) -> (-66.0671, 69.3641)
  line L98 (-66.0671, 69.3641) -> (-66.0671, 61.7728)
  line L99 (-66.0671, 61.7728) -> (-67.1058, 61.7728)
  line L100 (-67.1058, 61.7728) -> (-67.1058, 69.3641)
  line L101 (-52.6313, 69.3641) -> (-47.0967, 69.3641)
  line L102 (-47.0967, 69.3641) -> (-47.0967, 68.4339)
  line L103 (-47.0967, 68.4339) -> (-51.6287, 68.4339)
  line L104 (-51.6287, 68.4339) -> (-51.6287, 66.1292)
  line L105 (-51.6287, 66.1292) -> (-47.4378, 66.1292)
  line L106 (-47.4378, 66.1292) -> (-47.4378, 65.2507)
  line L107 (-47.4378, 65.2507) -> (-51.6287, 65.2507)
  line L108 (-51.6287, 65.2507) -> (-51.6287, 62.6772)
  line L109 (-51.6287, 62.6772) -> (-47.0192, 62.6772)
  line L110 (-47.0192, 62.6772) -> (-47.0192, 61.7728)
  line L111 (-47.0192, 61.7728) -> (-52.6313, 61.7728)
  line L112 (-52.6313, 61.7728) -> (-52.6313, 69.3641)
  spline S80 degree 3 poles (-32.8237, 65.8863) (-32.341, 65.8863) (-31.9597, 65.9824) (-31.6796, 66.1757) knots 0 0 0 0 1 1 1 1
  spline S81 degree 3 poles (-31.6796, 66.1757) (-31.3985, 66.3689) (-31.2579, 66.7162) (-31.2579, 67.2195) knots 0 0 0 0 1 1 1 1
  spline S82 degree 3 poles (-31.2579, 67.2195) (-31.2579, 67.7601) (-31.4543, 68.129) (-31.847, 68.3254) knots 0 0 0 0 1 1 1 1
  spline S83 degree 3 poles (-31.847, 68.3254) (-32.0568, 68.4288) (-32.3379, 68.4804) (-32.6893, 68.4804) knots 0 0 0 0 1 1 1 1
  line L113 (-32.6893, 68.4804) -> (-35.2008, 68.4804)
  line L114 (-35.2008, 68.4804) -> (-35.2008, 65.8863)
  line L115 (-35.2008, 65.8863) -> (-32.8237, 65.8863)
  line L116 (-36.2292, 69.3641) -> (-32.7152, 69.3641)
  spline S84 degree 3 poles (-32.7152, 69.3641) (-32.1364, 69.3641) (-31.6589, 69.2793) (-31.2837, 69.1109) knots 0 0 0 0 1 1 1 1
  spline S85 degree 3 poles (-31.2837, 69.1109) (-30.5706, 68.7874) (-30.214, 68.189) (-30.214, 67.3177) knots 0 0 0 0 1 1 1 1
  spline S86 degree 3 poles (-30.214, 67.3177) (-30.214, 66.863) (-30.3081, 66.4909) (-30.4951, 66.2015) knots 0 0 0 0 1 1 1 1
  spline S87 degree 3 poles (-30.4951, 66.2015) (-30.6833, 65.9121) (-30.9458, 65.6796) (-31.2837, 65.5039) knots 0 0 0 0 1 1 1 1
  spline S88 degree 3 poles (-31.2837, 65.5039) (-30.9871, 65.3829) (-30.7639, 65.2248) (-30.615, 65.0284) knots 0 0 0 0 1 1 1 1
  spline S89 degree 3 poles (-30.615, 65.0284) (-30.4652, 64.8321) (-30.3815, 64.5137) (-30.3639, 64.0724) knots 0 0 0 0 1 1 1 1
  line L117 (-30.3639, 64.0724) -> (-30.3277, 63.0544)
  spline S90 degree 3 poles (-30.3277, 63.0544) (-30.3174, 62.765) (-30.2936, 62.55) (-30.2554, 62.4084) knots 0 0 0 0 1 1 1 1
  spline S91 degree 3 poles (-30.2554, 62.4084) (-30.1934, 62.1676) (-30.0828, 62.0126) (-29.9246, 61.9434) knots 0 0 0 0 1 1 1 1
  line L118 (-29.9246, 61.9434) -> (-29.9246, 61.7728)
  line L119 (-29.9246, 61.7728) -> (-31.1855, 61.7728)
  spline S92 degree 3 poles (-31.1855, 61.7728) (-31.2197, 61.8379) (-31.2476, 61.9227) (-31.2682, 62.026) knots 0 0 0 0 1 1 1 1
  spline S93 degree 3 poles (-31.2682, 62.026) (-31.2889, 62.1294) (-31.3065, 62.3289) (-31.3199, 62.6255) knots 0 0 0 0 1 1 1 1
  line L120 (-31.3199, 62.6255) -> (-31.3819, 63.8916)
  spline S94 degree 3 poles (-31.3819, 63.8916) (-31.4057, 64.3877) (-31.5907, 64.7205) (-31.9349, 64.8889) knots 0 0 0 0 1 1 1 1